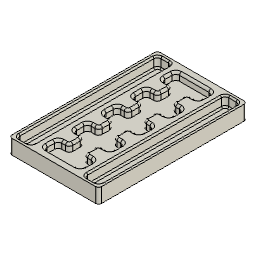
IOMOD-Cap (Autodesk Fusion 360 design; units mm, degrees)
Autodesk Fusion 360 part; units mm, degrees
sketch "Sketch1" plane through (0, 0, 0) normal (0, 0, 1) x (1, 0, 0)
  line L0 (6.1, -10.1) -> (-6.1, -10.1)
  line L1 (-6.1, -10.1) -> (-6.1, 10.1)
  line L2 (-6.1, 10.1) -> (6.1, 10.1)
  line L3 (6.1, 10.1) -> (6.1, -10.1)
  line L4 (6.1, -10.1) -> (-6.1, 10.1) construction
  line L5 (-6.1, -10.1) -> (6.1, 10.1) construction
  dimension "d1" = 12.2
  dimension "d2" = 20.2
  constraint horizontal L0
  constraint perpendicular L0 L1
  constraint parallel L0 L2
  constraint parallel L1 L3
  constraint coincident L4 origin
  constraint coincident L5 origin
  measures "d1" distance of L1.end L2.end
  measures "d2" distance of L0.end L1.end
extrude "Extrude1" add sketch "Sketch1" along normal blind 2
sketch "Sketch2" plane through (0, 0, 2) normal (0, 0, 1) x (-1, 0, 0)
  line L0 (-6.1, -10.1) -> (6.1, -10.1)
  line L1 (6.1, -10.1) -> (6.1, 10.1)
  line L2 (6.1, 10.1) -> (-6.1, 10.1)
  line L3 (-6.1, 10.1) -> (-6.1, -10.1)
  line L4 (4.1, 9.6) -> (5.1, 9.6)
  line L5 (5.6, 9.1) -> (5.6, -9.1)
  line L6 (5.1, -9.6) -> (4.1, -9.6)
  line L7 (3.6, -9.1) -> (3.6, 9.1)
  line L8 (3.6, 9.6) -> (5.6, -9.6) construction
  line L9 (5.6, 9.6) -> (3.6, -9.6) construction
  line L10 (-5.1, 9.6) -> (-4.1, 9.6)
  line L11 (-3.6, 9.1) -> (-3.6, -9.1)
  line L12 (-4.1, -9.6) -> (-5.1, -9.6)
  line L13 (-5.6, -9.1) -> (-5.6, 9.1)
  line L14 (-5.6, 9.6) -> (-3.6, -9.6) construction
  line L15 (-3.6, 9.6) -> (-5.6, -9.6) construction
  arc A0 (5.1, -9.6) -> (5.6, -9.1) centre (5.1, -9.1) ccw
  arc A1 (3.6, -9.1) -> (4.1, -9.6) centre (4.1, -9.1) ccw
  arc A2 (5.6, 9.1) -> (5.1, 9.6) centre (5.1, 9.1) ccw
  arc A3 (4.1, 9.6) -> (3.6, 9.1) centre (4.1, 9.1) ccw
  arc A4 (-5.6, -9.1) -> (-5.1, -9.6) centre (-5.1, -9.1) ccw
  arc A5 (-4.1, -9.6) -> (-3.6, -9.1) centre (-4.1, -9.1) ccw
  arc A6 (-3.6, 9.1) -> (-4.1, 9.6) centre (-4.1, 9.1) ccw
  arc A7 (-5.1, 9.6) -> (-5.6, 9.1) centre (-5.1, 9.1) ccw
  line L16 (-7, 0) -> (8, 0) construction
  line L17 (2.5, -1) -> (-2.5, -1)
  line L18 (-2.5, -1) -> (-2.5, 1)
  line L19 (-2.5, 1) -> (2.5, 1)
  line L20 (2.5, 1) -> (2.5, -1)
  line L21 (2.5, -1) -> (-2.5, 1) construction
  line L22 (-2.5, -1) -> (2.5, 1) construction
  line L23 (-2.5, -7) -> (2.5, -7)
  line L24 (2.5, -7) -> (2.5, -9)
  line L25 (2.5, -9) -> (-2.5, -9)
  line L26 (-2.5, -9) -> (-2.5, -7)
  line L27 (-2.5, -3) -> (2.5, -3)
  line L28 (2.5, -3) -> (2.5, -5)
  line L29 (2.5, -5) -> (-2.5, -5)
  line L30 (-2.5, -5) -> (-2.5, -3)
  line L31 (-2.5, 5) -> (2.5, 5)
  line L32 (2.5, 5) -> (2.5, 3)
  line L33 (2.5, 3) -> (-2.5, 3)
  line L34 (-2.5, 3) -> (-2.5, 5)
  line L35 (-2.5, 9) -> (2.5, 9)
  line L36 (2.5, 9) -> (2.5, 7)
  line L37 (2.5, 7) -> (-2.5, 7)
  line L38 (-2.5, 7) -> (-2.5, 9)
  line L39 (-1, 9) -> (1, 9)
  line L40 (1, 9) -> (1, -9)
  line L41 (1, -9) -> (-1, -9)
  line L42 (-1, -9) -> (-1, 9)
  line L43 (-1, 9) -> (1, -9) construction
  line L44 (1, 9) -> (-1, -9) construction
  point P0 (4.6, 0)
  point P1 (-4.6, 0)
  dimension "d5" = 2
  dimension "d6" = 19.2
  dimension "d7" = 2
  dimension "d8" = 19.2
  dimension "d9" = 0.5
  dimension "d10" = 0.5
  dimension "d11" = 0.5
  dimension "d12" = 0.5
  dimension "d13" = 0.5
  dimension "d14" = 0.5
  dimension "d15" = 0.5
  dimension "d16" = 0.5
  dimension "d17" = 0.5
  dimension "d18" = 0.5
  dimension "d27" = 9
  dimension "d28" = 8
  constraint horizontal L4
  constraint perpendicular L4 L5
  constraint parallel L4 L6
  constraint parallel L5 L7
  constraint coincident L8 P0
  constraint coincident L9 P0
  constraint horizontal L10
  constraint perpendicular L10 L11
  constraint parallel L10 L12
  constraint parallel L11 L13
  constraint coincident L14 P1
  constraint coincident L15 P1
  constraint coincident L8.end L5
  constraint coincident L8.end L6
  constraint tangent L5 A0
  constraint tangent L6 A0
  constraint coincident L9.end L6
  constraint coincident L9.end L7
  constraint tangent L6 A1
  constraint tangent L7 A1
  constraint coincident L9.start L4
  constraint coincident L9.start L5
  constraint tangent L4 A2
  constraint tangent L5 A2
  constraint coincident L8.start L4
  constraint coincident L8.start L7
  constraint tangent L4 A3
  constraint tangent L7 A3
  constraint coincident L15.end L12
  constraint coincident L15.end L13
  constraint tangent L12 A4
  constraint tangent L13 A4
  constraint coincident L14.end L12
  constraint coincident L14.end L11
  constraint tangent L12 A5
  constraint tangent L11 A5
  constraint coincident L15.start L11
  constraint coincident L15.start L10
  constraint tangent L11 A6
  constraint tangent L10 A6
  constraint coincident L14.start L13
  constraint coincident L14.start L10
  constraint tangent L13 A7
  constraint tangent L10 A7
  constraint perpendicular L3 L16
  constraint coincident P1 L16
  constraint coincident P0 L16
  constraint horizontal L17
  constraint perpendicular L17 L18
  constraint parallel L17 L19
  constraint parallel L18 L20
  constraint coincident L21 origin
  constraint coincident L22 origin
  constraint horizontal L39
  constraint perpendicular L39 L40
  constraint parallel L39 L41
  constraint parallel L40 L42
  constraint coincident L43 origin
  constraint coincident L44 origin
  constraint coincident L35 L39.start
  measures "d5" distance of L8.end L9.end
  measures "d6" distance of L9.start L8.end
  measures "d7" distance of L14.end L15.end
  measures "d8" distance of L15.start L14.end
  measures "d9" distance of L3 L13
  measures "d10" distance of L1 L5
  measures "d11" radius of A0
  measures "d12" radius of A1
  measures "d13" radius of A2
  measures "d14" radius of A3
  measures "d15" radius of A4
  measures "d16" radius of A5
  measures "d17" radius of A6
  measures "d18" radius of A7
extrude "Extrude2" cut sketch "Sketch2" against normal blind 1.4 contours L4 L5 L6 L7 A0 A1 A2 A3 | L10 L11 L12 L13 A4 A5 A6 A7
fillet "Fillet1" radius 0.4 4 edges at (6.1, -10.1, 1) (-6.1, -10.1, 1) (6.1, 10.1, 1) (-6.1, 10.1, 1)
fillet "Fillet2" radius 0.2 32 edges at (4.6, 9.6, 0.6) (5.4536, 9.4536, 0.6) (5.6, 0, 0.6) (5.4536, -9.4536, 0.6) (4.6, -9.6, 0.6) (3.7464, -9.4536, 0.6) (3.6, 0, 0.6) (3.7464, 9.4536, 0.6) (-4.6, 9.6, 0.6) (-3.7464, 9.4536, 0.6) (-3.6, 0, 0.6) (-3.7464, -9.4536, 0.6) (-4.6, -9.6, 0.6) (-5.4536, -9.4536, 0.6) (-5.6, 0, 0.6) (-5.4536, 9.4536, 0.6) (-4.6, -9.6, 2) (-5.4536, -9.4536, 2) (-5.6, 0, 2) (-5.4536, 9.4536, 2) (-4.6, 9.6, 2) (-3.7464, 9.4536, 2) (-3.6, 0, 2) (-3.7464, -9.4536, 2) (5.4536, 9.4536, 2) (5.6, 0, 2) (5.4536, -9.4536, 2) (4.6, -9.6, 2) (3.7464, -9.4536, 2) (3.6, 0, 2) (3.7464, 9.4536, 2) (4.6, 9.6, 2)
extrude "Extrude3" cut sketch "Sketch2" against normal blind 1 contours L17 L19 L20 L40 | L17 L27 L40 L42 | L17 L19 L40 L42 | L17 L18 L19 L42 | L19 L33 L40 L42 | L27 L29 L40 L42 | L27 L28 L29 L40 | L27 L29 L30 L42 | L31 L32 L33 L40 | L31 L33 L40 L42 | L23 L29 L40 L42 | L31 L33 L34 L42 | L31 L37 L40 L42 | L23 L25 L40 L41 L42 | L23 L24 L25 L40 | L23 L25 L26 L42 | L35 L36 L37 L40 | L35 L37 L39 L40 L42 | L35 L37 L38 L42
fillet "Fillet3" radius 0.5 20 edges at (-2.5, -9, 1.5) (-2.5, -5, 1.5) (-2.5, -1, 1.5) (-2.5, 3, 1.5) (-2.5, 7, 1.5) (2.5, -9, 1.5) (2.5, -5, 1.5) (2.5, -1, 1.5) (2.5, 3, 1.5) (2.5, 7, 1.5) (2.5, -7, 1.5) (2.5, -3, 1.5) (2.5, 1, 1.5) (2.5, 5, 1.5) (2.5, 9, 1.5) (-2.5, 9, 1.5) (-2.5, 5, 1.5) (-2.5, 1, 1.5) (-2.5, -3, 1.5) (-2.5, -7, 1.5)
fillet "Fillet4" radius 0.5 16 edges at (-1, 5, 1.5) (-1, 7, 1.5) (-1, 3, 1.5) (-1, 1, 1.5) (-1, -1, 1.5) (-1, -3, 1.5) (-1, -5, 1.5) (-1, -7, 1.5) (1, -7, 1.5) (1, -3, 1.5) (1, 1, 1.5) (1, 5, 1.5) (1, -5, 1.5) (1, -1, 1.5) (1, 3, 1.5) (1, 7, 1.5)
fillet "Fillet5" radius 0.3 72 edges at (2.3536, 8.8536, 2) (2.5, 8, 2) (2.3536, 7.1464, 2) (1.75, 7, 2) (1.1464, 6.8536, 2) (1, 6, 2) (1.1464, 5.1464, 2) (1.75, 5, 2) (2.3536, 4.8536, 2) (2.5, 4, 2) (2.3536, 3.1464, 2) (1.75, 3, 2) (1.1464, 2.8536, 2) (1, 2, 2) (1.1464, 1.1464, 2) (1.75, 1, 2) (2.3536, 0.8536, 2) (2.5, 0, 2) (2.3536, -0.8536, 2) (1.75, -1, 2) (1.1464, -1.1464, 2) (1, -2, 2) (1.1464, -2.8536, 2) (1.75, -3, 2) (2.3536, -3.1464, 2) (2.5, -4, 2) (2.3536, -4.8536, 2) (1.75, -5, 2) (1.1464, -5.1464, 2) (1, -6, 2) (1.1464, -6.8536, 2) (1.75, -7, 2) (2.3536, -7.1464, 2) (2.5, -8, 2) (2.3536, -8.8536, 2) (0, -9, 2) (-2.3536, -8.8536, 2) (-2.5, -8, 2) (-2.3536, -7.1464, 2) (-1.75, -7, 2) (-1.1464, -6.8536, 2) (-1, -6, 2) (-1.1464, -5.1464, 2) (-1.75, -5, 2) (-2.3536, -4.8536, 2) (-2.5, -4, 2) (-2.3536, -3.1464, 2) (-1.75, -3, 2) (-1.1464, -2.8536, 2) (-1, -2, 2) (-1.1464, -1.1464, 2) (-1.75, -1, 2) (-2.3536, -0.8536, 2) (-2.5, 0, 2) (-2.3536, 0.8536, 2) (-1.75, 1, 2) (-1.1464, 1.1464, 2) (-1, 2, 2) (-1.1464, 2.8536, 2) (-1.75, 3, 2) (-2.3536, 3.1464, 2) (-2.5, 4, 2) (-2.3536, 4.8536, 2) (-1.75, 5, 2) (-1.1464, 5.1464, 2) (-1, 6, 2) (-1.1464, 6.8536, 2) (-1.75, 7, 2) (-2.3536, 7.1464, 2) (-2.5, 8, 2) (-2.3536, 8.8536, 2) (0, 9, 2)
